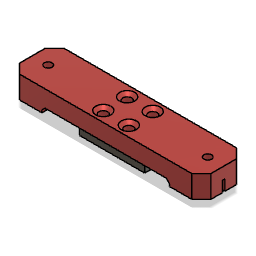
A shake table - slider mounting (Autodesk Fusion 360 design; units mm, degrees)
Autodesk Fusion 360 part; units mm, degrees
sketch "slider overall size" plane through (0, 0, 0) normal (0, 1, 0) x (1, 0, 0)
  line L0 (0, 0) -> (-41, 0)
  line L1 (-41, 0) -> (-41, -20)
  line L2 (-41, -20) -> (0, -20)
  line L3 (0, -20) -> (0, 0)
  dimension "d10" = 41
  dimension "d11" = 20
  constraint horizontal L0
  constraint vertical L1
  constraint horizontal L2
  constraint vertical L3
  constraint coincident L0.start L3.end
  measures "d10" distance of L0.start L0.end
  measures "d11" distance of L0.start L2.end
sketch "slider side" plane through (0, 0, 0) normal (1, 0, 0) x (0, 0, -1)
  line L0 (-20, 0) -> (-20, 8)
  line L1 (-20, 8) -> (0, 8)
  line L2 (0, 8) -> (0, 0)
  line L3 (-10, 11.4127) -> (-10, -6.2748) construction
  line L4 (-5.5, 0) -> (-5.5, 4.2)
  line L5 (-5.5, 4.2) -> (-10, 4.2)
  line L6 (0, 0) -> (-5.5, 0)
  line L7 (-10, 0) -> (-20, 0)
  line L8 (-14.5, 4.2) -> (-10, 4.2)
  line L9 (-14.5, 0) -> (-14.5, 4.2)
  line L10 (-20, 0) -> (-14.5, 0)
  dimension "d12" = 20
  dimension "d13" = 8
  dimension "d14" = 10
  dimension "d15" = 4.2
  dimension "d16" = 4.5
  dimension "d284" = 3.8
  constraint horizontal L6
  constraint vertical L0
  constraint horizontal L1
  constraint vertical L2
  constraint coincident L2.end L6.start
  constraint perpendicular L1 L3
  constraint perpendicular L4 L6
  constraint coincident L3 L5.end
  constraint perpendicular L4 L5
  constraint coincident L3 L7.start
  constraint collinear L6 L7
  constraint symmetric L2.end L3 L0.start
  constraint symmetric L3 L4.start L9.start
  constraint symmetric L3 L4.end L8.start
  constraint symmetric L3 L5.end L8.end
  measures "d12" distance of L2.end L0.start
  measures "d13" distance of L2.end L1.end
  measures "d14" distance of L3 L2.end
  measures "d15" distance of L4.start L4.end
  measures "d16" distance of L4.end L5.end
  measures "d20" diameter of L2.end
  measures "d254" diameter of L2.end
  measures "d255" diameter of L2.end
  measures "d284" distance of L1 L8
extrude "Extrude1" add sketch "slider side" against normal blind 41 makes body 1
sketch "slider screw holes" plane through (0, 8, 0) normal (0, 1, 0) x (-1, 0, 0)
  line L0 (0, 20) -> (0, 0)
  line L1 (0, 0) -> (41, 0)
  line L2 (41, 0) -> (41, 20)
  line L3 (41, 20) -> (0, 20)
  line L4 (20.5, 20) -> (20.5, 0)
  circle A0 centre (12.5, 17.5) radius 1.6
  line L5 (12.5, 18.1016) -> (12.5, 1.3766) construction
  line L6 (10, 17.5) -> (33.6736, 17.5) construction
  line L7 (0, 10) -> (41, 10)
  circle A1 centre (28.5, 17.5) radius 1.6
  circle A2 centre (12.5, 2.5) radius 1.6
  circle A3 centre (28.5, 2.5) radius 1.6
  dimension "d20" = 3.2
  dimension "d23" = 16
  dimension "d25" = 15
  constraint perpendicular L1 L4
  constraint perpendicular L3 L5
  constraint coincident A0.centre L5
  constraint perpendicular L4 L6
  constraint midpoint L3 L4.start
  constraint midpoint L1 L4.end
  constraint midpoint L0 L7.start
  constraint midpoint L2 L7.end
  constraint coincident A0.centre L6
  constraint symmetric L4 A0 A1
  constraint symmetric A0 L7 A2
  constraint symmetric L7 A1 A3
  measures "d20" diameter of A0
extrude "Extrude2" cut sketch "slider screw holes" against normal blind 4 contours A0 | A1 | A2 | A3 bodies 1
ref_plane "WorkPlane1" through (0, 8, 0) normal (0, 1, 0) x (0, 0, 1)
sketch "slider mount" plane through (0, 8, 0) normal (0, 1, 0) x (1, 0, 0)
  circle A0 centre (-12.5, -17.5) radius 1.6
  circle A1 centre (-12.5, -2.5) radius 1.6
  circle A2 centre (-28.5, -17.5) radius 1.6
  circle A3 centre (-28.5, -2.5) radius 1.6
  line L0 (0, -20) -> (0, 0)
  line L1 (0, 0) -> (-41, 0)
  line L2 (-41, 0) -> (-41, -20)
  line L3 (-41, -20) -> (0, -20)
  line L4 (0, -10) -> (-41, -10)
  line L5 (-20.5, -20) -> (-20.5, 0)
  line L6 (-80.5, 4) -> (39.5, 4)
  line L7 (39.5, 4) -> (39.5, -24)
  line L8 (39.5, -24) -> (-80.5, -24)
  line L9 (-80.5, -24) -> (-80.5, 4)
  circle A4 centre (-70.5, -10) radius 2.4
  circle A5 centre (29.5, -10) radius 2.4
  dimension "d248" = 4.8
  dimension "d249" = 100
  dimension "d252" = 10
  dimension "d253" = 14
  constraint midpoint L0 L4.start
  constraint midpoint L2 L4.end
  constraint midpoint L3 L5.start
  constraint midpoint L1 L5.end
  constraint horizontal L6
  constraint vertical L7
  constraint horizontal L8
  constraint vertical L9
  constraint symmetric L5 A4 A5
  constraint symmetric L4 L6 L8
  constraint symmetric L5 L7 L9
  constraint coincident L4 A4.centre
  measures "d248" diameter of A4
  measures "d249" distance of A4.centre A5.centre
  measures "d252" distance of L9 A4.centre
  measures "d253" distance of L6 A4.centre
extrude "Extrude3" add sketch "slider mount" along normal blind 10.5 separate body contours L0 L3 L4 L5 | L0 L1 L4 L5 | L2 L3 L4 L5 | L1 L2 L4 L5 | L6 L7 L8 L9 | A4 | A5 makes body 2
chamfer "Chamfer2" distance 6 angle 45 4 edges at (-80.5, 13.25, 24) (39.5, 13.25, 24) (39.5, 13.25, -4) (-80.5, 13.25, -4) on bodies 2
sketch "mount to slider holes" plane through (0, 18.5, 0) normal (0, 1, 0) x (-1, 0, 0)
  circle A0 centre (12.5, 17.5) radius 1.6
  circle A1 centre (28.5, 17.5) radius 1.6
  circle A2 centre (28.5, 2.5) radius 1.6
  circle A3 centre (12.5, 2.5) radius 1.6
  line L0 (74.5, -4) -> (80.5, 2)
  line L1 (80.5, 2) -> (80.5, 18)
  line L2 (80.5, 18) -> (74.5, 24)
  line L3 (74.5, 24) -> (-33.5, 24)
  line L4 (-33.5, 24) -> (-39.5, 18)
  line L5 (-39.5, 18) -> (-39.5, 2)
  line L6 (-39.5, 2) -> (-33.5, -4)
  line L7 (-33.5, -4) -> (74.5, -4)
  circle A4 centre (12.5, 2.5) radius 2.75
  circle A5 centre (12.5, 17.5) radius 2.75
  circle A6 centre (28.5, 17.5) radius 2.75
  circle A7 centre (28.5, 2.5) radius 2.75
  dimension "d254" = 5.5
  dimension "d255" = 5.5
  dimension "d256" = 5.5
  dimension "d257" = 5.5
  constraint concentric A3 A4
  constraint concentric A0 A5
  constraint concentric A1 A6
  constraint concentric A2 A7
  measures "d254" diameter of A4
  measures "d255" diameter of A5
  measures "d256" diameter of A6
  measures "d257" diameter of A7
extrude "Extrude27" cut sketch "mount to slider holes" against normal blind 6.3 contours A4 | A5 | A6 | A7 bodies 2
sketch "mount to belt dent" plane through (0, 8, 0) normal (0, -1, 0) x (1, 0, 0)
  line L0 (-80.5, 2) -> (-74.5, -4)
  line L1 (-74.5, -4) -> (33.5, -4)
  line L2 (33.5, -4) -> (39.5, 2)
  line L3 (39.5, 2) -> (39.5, 18)
  line L4 (39.5, 18) -> (33.5, 24)
  line L5 (33.5, 24) -> (-74.5, 24)
  line L6 (-74.5, 24) -> (-80.5, 18)
  line L7 (-80.5, 18) -> (-80.5, 2)
  circle A0 centre (-28.5, 17.5) radius 1.6
  circle A1 centre (-12.5, 17.5) radius 1.6
  circle A2 centre (-28.5, 2.5) radius 1.6
  circle A3 centre (-12.5, 2.5) radius 1.6
  line L8 (29.5, 10) -> (50, 10) construction
  line L9 (19.5, 9.25) -> (39.5, 9.25)
  line L10 (19.5, 24) -> (19.5, 10.75)
  line L11 (19.5, 9.25) -> (19.5, -4)
  arc A4 (19.9583, 10.5278) -> (20.8541, 10.5278) centre (20.4062, 10.75) ccw
  line L12 (20.4062, 10.75) -> (20.4062, 7.6132) construction
  line L13 (19.5, 10.75) -> (19.6, 10.75)
  arc A5 (21.2125, 10.75) -> (20.8541, 10.5278) centre (21.2125, 10.35) ccw
  arc A6 (19.9583, 10.5278) -> (19.6, 10.75) centre (19.6, 10.35) ccw
  line L14 (21.2125, 10.75) -> (21.6, 10.75)
  line L15 (21.6, 10.75) -> (39.5, 10.75) construction
  line L16 (23.2125, 10.75) -> (23.6, 10.75)
  arc A7 (23.2125, 10.75) -> (22.8541, 10.5278) centre (23.2125, 10.35) ccw
  arc A8 (21.9583, 10.5278) -> (22.8541, 10.5278) centre (22.4062, 10.75) ccw
  arc A9 (21.9583, 10.5278) -> (21.6, 10.75) centre (21.6, 10.35) ccw
  line L17 (25.2125, 10.75) -> (25.6, 10.75)
  arc A10 (25.2125, 10.75) -> (24.8541, 10.5278) centre (25.2125, 10.35) ccw
  arc A11 (23.9583, 10.5278) -> (24.8541, 10.5278) centre (24.4062, 10.75) ccw
  arc A12 (23.9583, 10.5278) -> (23.6, 10.75) centre (23.6, 10.35) ccw
  line L18 (27.2125, 10.75) -> (27.6, 10.75)
  arc A13 (27.2125, 10.75) -> (26.8541, 10.5278) centre (27.2125, 10.35) ccw
  arc A14 (25.9583, 10.5278) -> (26.8541, 10.5278) centre (26.4062, 10.75) ccw
  arc A15 (25.9583, 10.5278) -> (25.6, 10.75) centre (25.6, 10.35) ccw
  line L19 (29.2125, 10.75) -> (29.6, 10.75)
  arc A16 (29.2125, 10.75) -> (28.8541, 10.5278) centre (29.2125, 10.35) ccw
  arc A17 (27.9583, 10.5278) -> (28.8541, 10.5278) centre (28.4062, 10.75) ccw
  arc A18 (27.9583, 10.5278) -> (27.6, 10.75) centre (27.6, 10.35) ccw
  line L20 (31.2125, 10.75) -> (31.6, 10.75)
  arc A19 (31.2125, 10.75) -> (30.8541, 10.5278) centre (31.2125, 10.35) ccw
  arc A20 (29.9583, 10.5278) -> (30.8541, 10.5278) centre (30.4062, 10.75) ccw
  arc A21 (29.9583, 10.5278) -> (29.6, 10.75) centre (29.6, 10.35) ccw
  line L21 (33.2125, 10.75) -> (33.6, 10.75)
  arc A22 (33.2125, 10.75) -> (32.8541, 10.5278) centre (33.2125, 10.35) ccw
  arc A23 (31.9583, 10.5278) -> (32.8541, 10.5278) centre (32.4062, 10.75) ccw
  arc A24 (31.9583, 10.5278) -> (31.6, 10.75) centre (31.6, 10.35) ccw
  line L22 (35.2125, 10.75) -> (35.6, 10.75)
  arc A25 (35.2125, 10.75) -> (34.8541, 10.5278) centre (35.2125, 10.35) ccw
  arc A26 (33.9583, 10.5278) -> (34.8541, 10.5278) centre (34.4062, 10.75) ccw
  arc A27 (33.9583, 10.5278) -> (33.6, 10.75) centre (33.6, 10.35) ccw
  line L23 (37.2125, 10.75) -> (37.6, 10.75)
  arc A28 (37.2125, 10.75) -> (36.8541, 10.5278) centre (37.2125, 10.35) ccw
  arc A29 (35.9583, 10.5278) -> (36.8541, 10.5278) centre (36.4062, 10.75) ccw
  arc A30 (35.9583, 10.5278) -> (35.6, 10.75) centre (35.6, 10.35) ccw
  line L24 (39.2125, 10.75) -> (39.6, 10.75)
  arc A31 (39.2125, 10.75) -> (38.8541, 10.5278) centre (39.2125, 10.35) ccw
  arc A32 (37.9583, 10.5278) -> (38.8541, 10.5278) centre (38.4062, 10.75) ccw
  arc A33 (37.9583, 10.5278) -> (37.6, 10.75) centre (37.6, 10.35) ccw
  point P0 (20.4062, 10.25)
  dimension "d262" = 20
  dimension "d265" = 1.5
  dimension "d267" = 0.4
  dimension "d268" = 0.1
  dimension "d269" = 2
  dimension "d270" = 0.5
  dimension "d272" = 1
  dimension "d275" = 2
  dimension "d276" = 0
  dimension "d279" = 13.25
  dimension "d280" = 13.25
  constraint coincident L1 L11.end
  constraint perpendicular L1 L10
  constraint perpendicular L3 L8
  constraint perpendicular L3 L13
  constraint coincident L9.start L10
  constraint coincident L3 L9.end
  constraint perpendicular L3 L9
  constraint collinear L10 L11
  constraint coincident A4.centre L12.start
  constraint perpendicular L12 L13
  constraint tangent A4 A5
  constraint tangent A4 A6
  constraint tangent L13 A6
  constraint equal A5 A6
  constraint tangent A5 L14
  constraint midpoint A4 P0
  constraint coincident L3 L15.end
  constraint perpendicular L3 L15
  constraint coincident A5.start L15
  constraint coincident L5 L10.start
  measures "d262" distance of L3 L10
  measures "d265" distance of L9 L13
  measures "d267" radius of A5
  measures "d268" distance of L10.end L13.end
  measures "d269" distance of L13.end L14.end
  measures "d270" radius of A4
  measures "d272" distance of L9 P0
  measures "d279" distance of L10.start L10.end
  measures "d280" distance of L11.end L9.start
extrude "Extrude28" add sketch "mount to belt dent" along normal blind 3.5 contours L1 L2 L3 L9 L11 | L3 L4 L5 L10 A4 L13 A5 A6 L14 L16 A7 A8 A9 L17 A10 A11 A12 L18 A13 A14 A15 L19 A16 A17 A18 L20 A19 A20 A21 L21 A22 A23 A24 L22 A25 A26 A27 L23 A28 A29 A30 L24 A31 A32 A33 bodies 2
sketch "plan b" plane through (0, 0, -4) normal (0, 0, -1) x (-1, 0, 0)
  line L0 (74.5, 8) -> (74.5, 18.5)
  line L1 (74.5, 18.5) -> (-33.5, 18.5)
  line L2 (-33.5, 18.5) -> (-33.5, 4.5)
  line L3 (-33.5, 4.5) -> (-19.5, 4.5)
  line L4 (-19.5, 4.5) -> (-19.5, 8)
  line L5 (-19.5, 8) -> (74.5, 8)
  line L6 (-19.5, 8) -> (-39.5, 8)
  line L7 (-19.6, 8) -> (-19.5, 8)
  line L8 (-13.9019, 6.25) -> (-40.4019, 6.25) construction
  line L9 (-19.5, 4.5) -> (-33.5, 4.5)
  circle A0 centre (-27.5524, 6.25) radius 1.65
  dimension "d281" = 3.3
  constraint horizontal L8
  constraint coincident L8 A0.centre
  measures "d281" diameter of A0
ref_plane "WorkPlane6" through (-20.5, 4, 10) normal (1, 0, 0) x (0, 0, -1)
mirror "Mirror3" about plane through (-20.5, 4, 10) normal (1, 0, 0) of bodies 2 merged
sketch "belt dent amended" plane through (0, 4.5, 0) normal (0, -1, 0) x (1, 0, 0)
  line L0 (39.2125, 10.75) -> (39.5, 10.75)
  line L1 (39.5, 10.75) -> (39.5, 18)
  line L2 (39.5, 18) -> (33.5, 24)
  line L3 (33.5, 24) -> (19.5, 24)
  line L4 (19.5, 24) -> (19.5, 10.75)
  line L5 (19.5, 10.75) -> (19.6, 10.75)
  arc A0 (19.9583, 10.5278) -> (19.6, 10.75) centre (19.6, 10.35) ccw
  arc A1 (19.9583, 10.5278) -> (20.8541, 10.5278) centre (20.4062, 10.75) ccw
  arc A2 (21.2125, 10.75) -> (20.8541, 10.5278) centre (21.2125, 10.35) ccw
  line L6 (21.2125, 10.75) -> (21.6, 10.75)
  arc A3 (21.9583, 10.5278) -> (21.6, 10.75) centre (21.6, 10.35) ccw
  arc A4 (21.9583, 10.5278) -> (22.8541, 10.5278) centre (22.4062, 10.75) ccw
  arc A5 (23.2125, 10.75) -> (22.8541, 10.5278) centre (23.2125, 10.35) ccw
  line L7 (23.2125, 10.75) -> (23.6, 10.75)
  arc A6 (23.9583, 10.5278) -> (23.6, 10.75) centre (23.6, 10.35) ccw
  arc A7 (23.9583, 10.5278) -> (24.8541, 10.5278) centre (24.4062, 10.75) ccw
  arc A8 (25.2125, 10.75) -> (24.8541, 10.5278) centre (25.2125, 10.35) ccw
  line L8 (25.2125, 10.75) -> (25.6, 10.75)
  arc A9 (25.9583, 10.5278) -> (25.6, 10.75) centre (25.6, 10.35) ccw
  arc A10 (25.9583, 10.5278) -> (26.8541, 10.5278) centre (26.4062, 10.75) ccw
  arc A11 (27.2125, 10.75) -> (26.8541, 10.5278) centre (27.2125, 10.35) ccw
  line L9 (27.2125, 10.75) -> (27.6, 10.75)
  arc A12 (27.9583, 10.5278) -> (27.6, 10.75) centre (27.6, 10.35) ccw
  arc A13 (27.9583, 10.5278) -> (28.8541, 10.5278) centre (28.4062, 10.75) ccw
  arc A14 (29.2125, 10.75) -> (28.8541, 10.5278) centre (29.2125, 10.35) ccw
  line L10 (29.2125, 10.75) -> (29.6, 10.75)
  arc A15 (29.9583, 10.5278) -> (29.6, 10.75) centre (29.6, 10.35) ccw
  arc A16 (29.9583, 10.5278) -> (30.8541, 10.5278) centre (30.4062, 10.75) ccw
  arc A17 (31.2125, 10.75) -> (30.8541, 10.5278) centre (31.2125, 10.35) ccw
  line L11 (31.2125, 10.75) -> (31.6, 10.75)
  arc A18 (31.9583, 10.5278) -> (31.6, 10.75) centre (31.6, 10.35) ccw
  arc A19 (31.9583, 10.5278) -> (32.8541, 10.5278) centre (32.4062, 10.75) ccw
  arc A20 (33.2125, 10.75) -> (32.8541, 10.5278) centre (33.2125, 10.35) ccw
  line L12 (33.2125, 10.75) -> (33.6, 10.75)
  arc A21 (33.9583, 10.5278) -> (33.6, 10.75) centre (33.6, 10.35) ccw
  arc A22 (33.9583, 10.5278) -> (34.8541, 10.5278) centre (34.4062, 10.75) ccw
  arc A23 (35.2125, 10.75) -> (34.8541, 10.5278) centre (35.2125, 10.35) ccw
  line L13 (35.2125, 10.75) -> (35.6, 10.75)
  arc A24 (35.9583, 10.5278) -> (35.6, 10.75) centre (35.6, 10.35) ccw
  arc A25 (35.9583, 10.5278) -> (36.8541, 10.5278) centre (36.4062, 10.75) ccw
  arc A26 (37.2125, 10.75) -> (36.8541, 10.5278) centre (37.2125, 10.35) ccw
  line L14 (37.2125, 10.75) -> (37.6, 10.75)
  arc A27 (37.9583, 10.5278) -> (37.6, 10.75) centre (37.6, 10.35) ccw
  arc A28 (37.9583, 10.5278) -> (38.8541, 10.5278) centre (38.4062, 10.75) ccw
  arc A29 (39.2125, 10.75) -> (38.8541, 10.5278) centre (39.2125, 10.35) ccw
  line L15 (19.5, 9.25) -> (19.5, -4)
  line L16 (19.5, -4) -> (33.5, -4)
  line L17 (33.5, -4) -> (39.5, 2)
  line L18 (39.5, 2) -> (39.5, 9.25)
  line L19 (39.5, 9.25) -> (19.5, 9.25)
  line L20 (-74.5, -4) -> (-80.5, 2)
  line L21 (-80.5, 2) -> (-80.5, 18)
  line L22 (-80.5, 18) -> (-74.5, 24)
  line L23 (-74.5, 24) -> (33.5, 24)
  line L24 (33.5, 24) -> (39.5, 18)
  line L25 (39.5, 18) -> (39.5, 2)
  line L26 (39.5, 2) -> (33.5, -4)
  line L27 (33.5, -4) -> (-74.5, -4)
  arc A30 (27.2202, 9.25) -> (31.7798, 9.25) centre (29.5, 10) ccw
  line L28 (27.2202, 9.25) -> (31.7798, 9.25)
  line L29 (39.5, 10.75) -> (39.5, 9.25)
  line L30 (19.5, 10.75) -> (19.5, 9.25)
  arc A31 (-25.75, 2.5) -> (-31.25, 2.5) centre (-28.5, 2.5) ccw
  arc A32 (-31.25, 2.5) -> (-25.75, 2.5) centre (-28.5, 2.5) ccw
  arc A33 (-25.75, 17.5) -> (-31.25, 17.5) centre (-28.5, 17.5) ccw
  arc A34 (-31.25, 17.5) -> (-25.75, 17.5) centre (-28.5, 17.5) ccw
  arc A35 (-9.75, 2.5) -> (-15.25, 2.5) centre (-12.5, 2.5) ccw
  arc A36 (-15.25, 2.5) -> (-9.75, 2.5) centre (-12.5, 2.5) ccw
  arc A37 (-9.75, 17.5) -> (-15.25, 17.5) centre (-12.5, 17.5) ccw
  arc A38 (-15.25, 17.5) -> (-9.75, 17.5) centre (-12.5, 17.5) ccw
  constraint coincident L0.end L1.start
  constraint coincident L18.end L19.start
  constraint coincident L4.end L5.start
  constraint coincident L15.start L19.end
extrude "Extrude29" cut sketch "belt dent amended" against normal blind 6.7 contours L0 L5 A0 A1 A2 L6 A3 A4 A5 L7 A6 A7 A8 L8 A9 A10 A11 L9 A12 A13 A14 L10 A15 A16 A17 L11 A18 A19 A20 L12 A21 A22 A23 L13 A24 A25 A26 L14 A27 A28 A29 L19 L25 L28 L29 L30 bodies 2
sketch "ROOM FOR BELT BENT FASTEN" plane through (0, 8, 0) normal (0, -1, 0) x (1, 0, 0)
  line L0 (19.5, 9.25) -> (19.5, 10.75)
  line L1 (19.5, 10.75) -> (19.5, 24)
  line L2 (19.5, 24) -> (-60.5, 24)
  line L3 (-60.5, 24) -> (-60.5, 10.75)
  line L4 (-60.5, 10.75) -> (-60.6, 10.75)
  arc A0 (-60.6, 10.75) -> (-60.9583, 10.5278) centre (-60.6, 10.35) ccw
  arc A1 (-61.8541, 10.5278) -> (-60.9583, 10.5278) centre (-61.4062, 10.75) ccw
  arc A2 (-61.8541, 10.5278) -> (-62.2125, 10.75) centre (-62.2125, 10.35) ccw
  line L5 (-62.2125, 10.75) -> (-62.6, 10.75)
  arc A3 (-62.6, 10.75) -> (-62.9583, 10.5278) centre (-62.6, 10.35) ccw
  arc A4 (-63.8541, 10.5278) -> (-62.9583, 10.5278) centre (-63.4062, 10.75) ccw
  arc A5 (-63.8541, 10.5278) -> (-64.2125, 10.75) centre (-64.2125, 10.35) ccw
  line L6 (-64.2125, 10.75) -> (-64.6, 10.75)
  arc A6 (-64.6, 10.75) -> (-64.9583, 10.5278) centre (-64.6, 10.35) ccw
  arc A7 (-65.8541, 10.5278) -> (-64.9583, 10.5278) centre (-65.4062, 10.75) ccw
  arc A8 (-65.8541, 10.5278) -> (-66.2125, 10.75) centre (-66.2125, 10.35) ccw
  line L7 (-66.2125, 10.75) -> (-66.6, 10.75)
  arc A9 (-66.6, 10.75) -> (-66.9583, 10.5278) centre (-66.6, 10.35) ccw
  arc A10 (-67.8541, 10.5278) -> (-66.9583, 10.5278) centre (-67.4062, 10.75) ccw
  arc A11 (-67.8541, 10.5278) -> (-68.2125, 10.75) centre (-68.2125, 10.35) ccw
  line L8 (-68.2125, 10.75) -> (-68.6, 10.75)
  line L9 (-80.5, 9.25) -> (-60.5, 9.25)
  line L10 (-60.5, 9.25) -> (-60.5, -4)
  line L11 (-60.5, -4) -> (19.5, -4)
  line L12 (19.5, -4) -> (19.5, 9.25)
  circle A12 centre (-28.5, 2.5) radius 1.6
  circle A13 centre (-12.5, 17.5) radius 1.6
  circle A14 centre (-12.5, 2.5) radius 1.6
  circle A15 centre (-28.5, 17.5) radius 1.6
  line L13 (19.5, 9.25) -> (19.5, -4)
  line L14 (19.5, -4) -> (33.5, -4)
  line L15 (33.5, -4) -> (39.5, 2)
  line L16 (39.5, 2) -> (39.5, 9.25)
  line L17 (39.5, 9.25) -> (19.5, 9.25)
  line L18 (39.2125, 10.75) -> (39.5, 10.75)
  line L19 (39.5, 10.75) -> (39.5, 18)
  line L20 (39.5, 18) -> (33.5, 24)
  line L21 (33.5, 24) -> (19.5, 24)
  line L22 (19.5, 24) -> (19.5, 10.75)
  line L23 (19.5, 10.75) -> (19.6, 10.75)
  arc A16 (19.9583, 10.5278) -> (19.6, 10.75) centre (19.6, 10.35) ccw
  arc A17 (19.9583, 10.5278) -> (20.8541, 10.5278) centre (20.4062, 10.75) ccw
  arc A18 (21.2125, 10.75) -> (20.8541, 10.5278) centre (21.2125, 10.35) ccw
  line L24 (21.2125, 10.75) -> (21.6, 10.75)
  arc A19 (21.9583, 10.5278) -> (21.6, 10.75) centre (21.6, 10.35) ccw
  arc A20 (21.9583, 10.5278) -> (22.8541, 10.5278) centre (22.4062, 10.75) ccw
  arc A21 (23.2125, 10.75) -> (22.8541, 10.5278) centre (23.2125, 10.35) ccw
  line L25 (23.2125, 10.75) -> (23.6, 10.75)
  arc A22 (23.9583, 10.5278) -> (23.6, 10.75) centre (23.6, 10.35) ccw
  arc A23 (23.9583, 10.5278) -> (24.8541, 10.5278) centre (24.4062, 10.75) ccw
  arc A24 (25.2125, 10.75) -> (24.8541, 10.5278) centre (25.2125, 10.35) ccw
  line L26 (25.2125, 10.75) -> (25.6, 10.75)
  arc A25 (25.9583, 10.5278) -> (25.6, 10.75) centre (25.6, 10.35) ccw
  arc A26 (25.9583, 10.5278) -> (26.8541, 10.5278) centre (26.4062, 10.75) ccw
  arc A27 (27.2125, 10.75) -> (26.8541, 10.5278) centre (27.2125, 10.35) ccw
  line L27 (27.2125, 10.75) -> (27.6, 10.75)
  arc A28 (27.9583, 10.5278) -> (27.6, 10.75) centre (27.6, 10.35) ccw
  arc A29 (27.9583, 10.5278) -> (28.8541, 10.5278) centre (28.4062, 10.75) ccw
  arc A30 (29.2125, 10.75) -> (28.8541, 10.5278) centre (29.2125, 10.35) ccw
  line L28 (29.2125, 10.75) -> (29.6, 10.75)
  arc A31 (29.9583, 10.5278) -> (29.6, 10.75) centre (29.6, 10.35) ccw
  arc A32 (29.9583, 10.5278) -> (30.8541, 10.5278) centre (30.4062, 10.75) ccw
  arc A33 (31.2125, 10.75) -> (30.8541, 10.5278) centre (31.2125, 10.35) ccw
  line L29 (31.2125, 10.75) -> (31.6, 10.75)
  arc A34 (31.9583, 10.5278) -> (31.6, 10.75) centre (31.6, 10.35) ccw
  arc A35 (31.9583, 10.5278) -> (32.8541, 10.5278) centre (32.4062, 10.75) ccw
  arc A36 (33.2125, 10.75) -> (32.8541, 10.5278) centre (33.2125, 10.35) ccw
  line L30 (33.2125, 10.75) -> (33.6, 10.75)
  arc A37 (33.9583, 10.5278) -> (33.6, 10.75) centre (33.6, 10.35) ccw
  arc A38 (33.9583, 10.5278) -> (34.8541, 10.5278) centre (34.4062, 10.75) ccw
  arc A39 (35.2125, 10.75) -> (34.8541, 10.5278) centre (35.2125, 10.35) ccw
  line L31 (35.2125, 10.75) -> (35.6, 10.75)
  arc A40 (35.9583, 10.5278) -> (35.6, 10.75) centre (35.6, 10.35) ccw
  arc A41 (35.9583, 10.5278) -> (36.8541, 10.5278) centre (36.4062, 10.75) ccw
  arc A42 (37.2125, 10.75) -> (36.8541, 10.5278) centre (37.2125, 10.35) ccw
  line L32 (37.2125, 10.75) -> (37.6, 10.75)
  arc A43 (37.9583, 10.5278) -> (37.6, 10.75) centre (37.6, 10.35) ccw
  arc A44 (37.9583, 10.5278) -> (38.8541, 10.5278) centre (38.4062, 10.75) ccw
  arc A45 (39.2125, 10.75) -> (38.8541, 10.5278) centre (39.2125, 10.35) ccw
  line L33 (39.5, 9.25) -> (39.5, 10.75) construction
  line L34 (39.5, 10) -> (2.5, 10) construction
  line L35 (19.5, 11.6) -> (5.5, 11.6)
  line L36 (5.5, 11.6) -> (5.5, 8.4)
  line L37 (5.5, 8.4) -> (19.5, 8.4)
  line L38 (19.5, 8.4) -> (19.5, 11.6)
  arc A46 (-68.6, 10.75) -> (-68.9583, 10.5278) centre (-68.6, 10.35) ccw
  arc A47 (-69.8541, 10.5278) -> (-68.9583, 10.5278) centre (-69.4062, 10.75) ccw
  arc A48 (-69.8541, 10.5278) -> (-70.2125, 10.75) centre (-70.2125, 10.35) ccw
  line L39 (-70.2125, 10.75) -> (-70.6, 10.75)
  arc A49 (-70.6, 10.75) -> (-70.9583, 10.5278) centre (-70.6, 10.35) ccw
  arc A50 (-71.8541, 10.5278) -> (-70.9583, 10.5278) centre (-71.4062, 10.75) ccw
  arc A51 (-71.8541, 10.5278) -> (-72.2125, 10.75) centre (-72.2125, 10.35) ccw
  line L40 (-72.2125, 10.75) -> (-72.6, 10.75)
  arc A52 (-72.6, 10.75) -> (-72.9583, 10.5278) centre (-72.6, 10.35) ccw
  arc A53 (-73.8541, 10.5278) -> (-72.9583, 10.5278) centre (-73.4062, 10.75) ccw
  arc A54 (-73.8541, 10.5278) -> (-74.2125, 10.75) centre (-74.2125, 10.35) ccw
  line L41 (-74.2125, 10.75) -> (-74.6, 10.75)
  arc A55 (-74.6, 10.75) -> (-74.9583, 10.5278) centre (-74.6, 10.35) ccw
  arc A56 (-75.8541, 10.5278) -> (-74.9583, 10.5278) centre (-75.4062, 10.75) ccw
  arc A57 (-75.8541, 10.5278) -> (-76.2125, 10.75) centre (-76.2125, 10.35) ccw
  line L42 (-76.2125, 10.75) -> (-76.6, 10.75)
  arc A58 (-76.6, 10.75) -> (-76.9583, 10.5278) centre (-76.6, 10.35) ccw
  arc A59 (-77.8541, 10.5278) -> (-76.9583, 10.5278) centre (-77.4062, 10.75) ccw
  arc A60 (-77.8541, 10.5278) -> (-78.2125, 10.75) centre (-78.2125, 10.35) ccw
  line L43 (-78.2125, 10.75) -> (-78.6, 10.75)
  arc A61 (-78.6, 10.75) -> (-78.9583, 10.5278) centre (-78.6, 10.35) ccw
  arc A62 (-79.8541, 10.5278) -> (-78.9583, 10.5278) centre (-79.4062, 10.75) ccw
  arc A63 (-79.8541, 10.5278) -> (-80.2125, 10.75) centre (-80.2125, 10.35) ccw
  line L44 (-80.2125, 10.75) -> (-80.5, 10.75)
  line L45 (-80.5, 10.75) -> (-80.5, 9.25)
  dimension "d287" = 3.2
  dimension "d288" = 14
  constraint coincident L16.end L17.start
  constraint coincident L18.end L19.start
  constraint midpoint L33 L34.start
  constraint perpendicular L33 L34
  constraint horizontal L35
  constraint vertical L36
  constraint horizontal L37
  constraint vertical L38
  constraint coincident L22 L35.start
  constraint symmetric L34 L35 L37
  measures "d287" distance of L35 L37
  measures "d288" distance of L22 L36
extrude "Extrude30" cut sketch "ROOM FOR BELT BENT FASTEN" against normal blind 3 contours L0 L1 L12 L13 L22 L35 L36 L37 L38 bodies 2
fillet "Fillet24" radius 0.4 2 edges at (5.5, 9.5, 8.4) (5.5, 9.5, 11.6) on bodies 2
chamfer "Chamfer4" distance 2 angle 45 2 edges at (19.5, 8, 17.8) (19.5, 8, 2.2) on bodies 2
mirror "Mirror4" about plane through (-20.5, 4, 10) normal (1, 0, 0) of bodies 2 makes body 3
sketch "Sketch35" plane through (0, 18.5, 0) normal (0, 1, 0) x (-1, 0, 0)
  line L0 (-39.5, 2) -> (-33.5, -4)
  line L1 (-33.5, -4) -> (74.5, -4)
  line L2 (74.5, -4) -> (80.5, 2)
  line L3 (80.5, 2) -> (80.5, 18)
  line L4 (80.5, 18) -> (74.5, 24)
  line L5 (74.5, 24) -> (-33.5, 24)
  line L6 (-33.5, 24) -> (-39.5, 18)
  line L7 (-39.5, 18) -> (-39.5, 2)
  circle A0 centre (-29.5, 10) radius 2.4
  circle A1 centre (70.5, 10) radius 2.4
  arc A2 (15.25, 2.5) -> (9.75, 2.5) centre (12.5, 2.5) ccw
  arc A3 (9.75, 2.5) -> (15.25, 2.5) centre (12.5, 2.5) ccw
  arc A4 (15.25, 17.5) -> (9.75, 17.5) centre (12.5, 17.5) ccw
  arc A5 (9.75, 17.5) -> (15.25, 17.5) centre (12.5, 17.5) ccw
  arc A6 (31.25, 2.5) -> (25.75, 2.5) centre (28.5, 2.5) ccw
  arc A7 (25.75, 2.5) -> (31.25, 2.5) centre (28.5, 2.5) ccw
  arc A8 (31.25, 17.5) -> (25.75, 17.5) centre (28.5, 17.5) ccw
  arc A9 (25.75, 17.5) -> (31.25, 17.5) centre (28.5, 17.5) ccw
extrude "Extrude31" cut sketch "Sketch35" against normal blind 4 contours A0 | A1 bodies 3
split "Split1" by plane through (-20.5, 4, 10) normal (1, 0, 0) bodies 3 makes body 4 at (2.4519, 18.5, 10)
mirror "Mirror5" about plane through (-20.5, 4, 10) normal (1, 0, 0) of bodies 3 merged
chamfer "Chamfer5" distance 2 angle 45 4 edges at (-9.9361, 18.5, 18.4944) (-9.9361, 18.5, 3.4944) (-31.0639, 18.5, 18.4944) (-31.0639, 18.5, 3.4944) on bodies 3
hidden bodies 2 4
equation "NumTeeth = 20"
equation "TeethPitch = 2 mm"
equation "PulleyDia = NumTeeth * TeethPitch"
equation "ToothAng = ( 360 / NumTeeth ) * 1 deg"
equation "TransOffsetAngle = ToothAng * 0.2"
equation "ShoulderRadius = 0.15 mm"
equation "RootRadius = 0.555 mm"
equation "TransRadius = 1 mm"
equation "ToothHeight = 0.75 mm"
equation "beltThickness = 1.5 mm"
equation "pulleyDia = 20.5 mm"
equation "pulleyDiaHalf = pulleyDia / 2"
equation "bridgeWidth = 10 mm"
equation "d254 = M3x8headdia"
equation "d255 = M3x8headdia"
equation "d256 = M3x8headdia"
equation "d257 = M3x8headdia"
equation "M3x8headdia = 5.5 mm"
named bodies: "linear rail slider", "sliderMount", "sliderMount - FINAL.....", "sliderMount (1) (1)"
